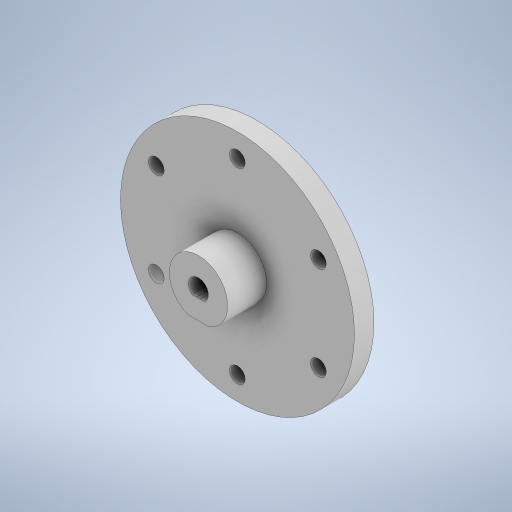
# Autodesk Inventor part: Radaufhängung_06
Saved by Autodesk Inventor 2024 (Build 280153000, 153)
## iProperties
Created: 2024-04-29
Part Number: Radaufhängung_06
Material: Generisch
Document SubType Name: Modeling
Designer: month
Density: 1 g/cm^3
Appearance: Vorgabe
Author: month
Autodesk Inventor part; units mm, degrees
ref_plane "YZ Plane" through (0, 0, 0) normal (1, 0, 0) x (0, 1, 0)
ref_plane "XZ Plane" through (0, 0, 0) normal (0, 1, 0) x (-1, 0, 0)
ref_plane "XY Plane" through (0, 0, 0) normal (0, 0, 1) x (1, 0, 0)
sketch "Skizze2" plane through (0, 0, 0) normal (0, 1, 0) x (-1, 0, 0)
  circle A0 centre (0, 0) radius 30
  dimension "d3" = 60
  constraints: 1 centre point, 1 coincident
  measures "d3" diameter of A0
extrude "Extrusion2" add sketch "Skizze2" along normal blind 5
sketch "Skizze3" plane through (0, 5, 0) normal (0, 1, 0) x (1, 0, 0)
  circle A0 centre (0, 0) radius 10.5
  dimension "d6" = 21
  constraints: 1 centre point, 1 coincident
  measures "d6" diameter of A0
extrude "Extrusion3" add sketch "Skizze3" along normal blind 7
sketch "Skizze4" plane through (0, 0, 0) normal (0, -1, 0) x (1, 0, 0)
  circle A0 centre (0, 0) radius 7.5
  dimension "d9" = 15
  constraints: 1 centre point, 1 coincident
  measures "d9" diameter of A0
extrude "Extrusion4" add sketch "Skizze4" along normal blind 10
sketch "Skizze5" plane through (0, -10, 0) normal (0, -1, 0) x (1, 0, 0)
  arc A0 (1.6432, -1.95) -> (-1.6432, -1.95) centre (0, 0) ccw
  line L0 (1.6432, -1.95) -> (-1.6432, -1.95)
  dimension "d12" = 5.1
  dimension "d14" = 4.5
  constraints: 2 end point, 2 point on circle, 1 centre point, 1 coincident, 1 horizontal
  measures "d12" diameter of A0
extrude "Extrusion5" cut sketch "Skizze5" against normal blind 20
sketch "Skizze6" plane through (-1.6432, -10, -1.95) normal (0, 0, 1) x (1, 0, 0)
  line L0 (-5.8568, 0) -> (9.1432, 0) projected
  line L1 (1.6432, 0) -> (1.6432, 10)
  line L2 (1.6432, 10) -> (1.6432, 0)
  circle A0 centre (1.6432, 5) radius 1
  dimension "d17" = 2
  dimension "d20" = 5
  constraints: 4 end point, 2 midpoint, 1 centre point, 1 collinear, 1 vertical
  measures "d17" diameter of A0
  measures "d20" distance from line of L0 A0.centre
extrude "Extrusion6" cut sketch "Skizze6" against normal blind 20
sketch "Skizze7" plane through (0, -10, 0) normal (0, -1, 0) x (1, 0, 0)
  circle A0 centre (0, 0) radius 7.5 projected
  line L0 (2.6926, -7) -> (-2.6926, -7)
  point P0 (0, -7)
  dimension "d23" = 7
  constraints: 2 end point, 2 point on circle, 1 horizontal, 1 midpoint
  measures "d23" distance of point (0, 0) point (0, -7)
extrude "Extrusion7" cut sketch "Skizze7" against normal blind 15 contours L0 A0 picked at (0.3052, -7.148)
sketch "Skizze8" plane through (0, 0, 0) normal (0, -1, 0) x (1, 0, 0)
  circle A0 centre (0, 0) radius 24 construction
  line L0 (20.7846, 12) -> (20.7846, -12) construction
  line L1 (20.7846, -12) -> (0, -24) construction
  line L2 (0, -24) -> (-20.7846, -12) construction
  line L3 (-20.7846, -12) -> (-20.7846, 12) construction
  line L4 (-20.7846, 12) -> (0, 24) construction
  line L5 (0, 24) -> (20.7846, 12) construction
  circle A1 centre (0, 0) radius 30 projected
  line L6 (30, 0) -> (-30, 0)
  line L7 (0, -30) -> (0, 30)
  circle A2 centre (0, -24) radius 2
  circle A3 centre (20.7846, -12) radius 2
  circle A4 centre (20.7846, 12) radius 2
  circle A5 centre (0, 24) radius 2
  circle A6 centre (-20.7846, 12) radius 2
  circle A7 centre (-20.7846, -12) radius 2
  dimension "d26" = 48
  dimension "d27" = 24
  dimension "d28" = 4
  dimension "d29" = 4
  dimension "d30" = 4
  dimension "d31" = 4
  dimension "d32" = 4
  dimension "d33" = 4
  constraints: 16 end point, 10 point on circle, 7 centre point, 7 coincident, 4 midpoint, 3 symmetric about line, 1 horizontal, 1 parallel, 1 perpendicular, 1 point on line, 1 vertical, 1 other
  measures "d26" diameter of A0
  measures "d27" distance of L2.end L3.end
  measures "d28" diameter of A3
  measures "d29" diameter of A2
  measures "d30" diameter of A4
  measures "d31" diameter of A5
  measures "d32" diameter of A6
  measures "d33" diameter of A7
extrude "Extrusion8" cut sketch "Skizze8" against normal blind 20 contours A5 L7 | L7 A5 | A2 L7 | L7 A2 | A3 | A4 | A6 | A7
sketch "Skizze9" plane through (0, 12, 0) normal (0, 1, 0) x (1, 0, 0)
  arc A0 (-1.6432, 1.95) -> (1.6432, 1.95) centre (0, 0) ccw projected
  circle A1 centre (0, 0) radius 8.5
  dimension "d36" = 17
  constraints: 1 centre point, 1 coincident
  measures "d36" diameter of A1
extrude "Extrusion9" add sketch "Skizze9" along normal blind 7.5
sketch "Skizze11" plane through (0, 19.5, 0) normal (0, 1, 0) x (1, 0, 0)
  circle A0 centre (0, 0) radius 2
  dimension "d47" = 4
  constraints: 1 centre point, 1 coincident
  measures "d47" diameter of A0
extrude "Extrusion10" cut sketch "Skizze11" against normal blind 50
